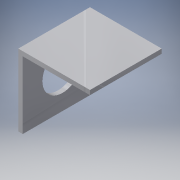
# Autodesk Inventor part: Lbracket
Saved by Autodesk Inventor 2016 (Build 200138000, 138)
## iProperties
Created: 2016-02-04
Part Number: Lbracket
Material: Aluminum 6061
Document SubType Name: Modeling
Designer: zachary
Density: 2.7 g/cm^3
Appearance: Aluminum - Flat
Mass: 37.3649 g
Surface Area: 99.4998 cm^2
Volume: 13.8388 cm^3
User Status: complete
Author: zachary
Autodesk Inventor part; units mm, degrees
ref_plane "YZ Plane" through (0, 0, 0) normal (1, 0, 0) x (0, 1, 0)
ref_plane "XZ Plane" through (0, 0, 0) normal (0, 1, 0) x (-1, 0, 0)
ref_plane "XY Plane" through (0, 0, 0) normal (0, 0, 1) x (1, 0, 0)
sketch "Sketch1" plane through (0, 0, 0) normal (0, 0, 1) x (1, 0, 0)
  line L0 (0, 0) -> (50.8, 0)
  line L1 (50.8, 0) -> (50.8, -3.175)
  line L2 (3.175, -50.8) -> (0, -50.8)
  line L3 (0, -50.8) -> (0, 0)
  line L4 (3.175, -50.8) -> (3.175, -3.175)
  line L5 (3.175, -3.175) -> (50.8, -3.175)
  dimension "d0" = 50.8
  dimension "d1" = 50.8
  dimension "d2" = 3.175
  dimension "d3" = 3.175
  constraints: 12 end point, 2 parallel, 1 horizontal, 1 perpendicular
  measures "d0" distance between parallel lines of L1 L3
  measures "d1" distance between parallel lines of L0 L2
  measures "d2" distance between parallel lines of L0 L5
  measures "d3" distance between parallel lines of L3 L4
extrude "Extrusion1" add sketch "Sketch1" along normal blind 50.8
sketch "Sketch2" plane through (0, -50.8, 0) normal (-1, 0, 0) x (0, 0, 1)
  circle A0 centre (22.5814, 25.4) radius 14.2875
  line L0 (0, 50.8) -> (50.8, 50.8) projected
  line L1 (0, 0) -> (50.8, 0) projected
  dimension "d6" = 25.4
  dimension "d7" = 25.4
  dimension "d8" = 28.575
  constraints: 1 centre point
  measures "d6" distance from line of L0 A0.centre
  measures "d7" distance from line of L1 A0.centre
  measures "d8" diameter of A0
extrude "Extrusion2" cut sketch "Sketch2" against normal through all
body "Solid1"
